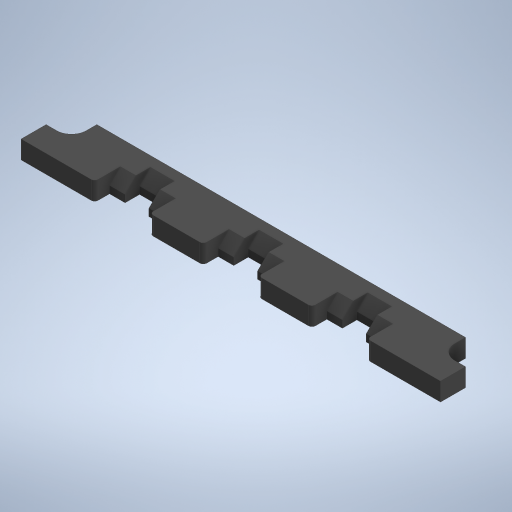
# Autodesk Inventor part: Centreur_resistance
Saved by Autodesk Inventor 2024 (Build 280153000, 153)
## iProperties
Created: 2024-08-30
Part Number: Centreur_resistance
Material: Générique
Document SubType Name: Modeling
Designer: malam
Density: 1 g/cm^3
Appearance: Par défaut
Author: malam
Autodesk Inventor part; units mm, degrees
ref_plane "YZ Plane" through (0, 0, 0) normal (1, 0, 0) x (0, 1, 0)
ref_plane "XZ Plane" through (0, 0, 0) normal (0, 1, 0) x (-1, 0, 0)
ref_plane "XY Plane" through (0, 0, 0) normal (0, 0, 1) x (1, 0, 0)
sketch "Esquisse1" plane through (0, 0, 0) normal (0, 1, 0) x (-1, 0, 0)
  line L0 (60, -42) -> (60, 42)
  line L1 (55, 39) -> (57, 39)
  arc A0 (52, 42) -> (55, 39) centre (55, 42) ccw
  line L2 (52, 44) -> (52, 42)
  line L3 (55, 46) -> (-55, 46)
  circle A1 centre (55, 42.115) radius 2
  arc A2 (60, 42) -> (55, 47) centre (55, 42) ccw
  line L4 (55, 47) -> (-55, 47)
  line L5 (-55, 47) -> (55, 47)
  line L6 (51, 45) -> (-51, 45)
  line L7 (-52, 42) -> (-51, 42)
  arc A3 (-57, 39) -> (-58, 38) centre (-57, 38) ccw
  circle A4 centre (-55, 42.115) radius 2
  line L8 (-55, 39) -> (-55, 38)
  line L9 (-52, 44) -> (-52, 42)
  arc A5 (-51, 45) -> (-52, 44) centre (-51, 44) ccw
  line L10 (-55, 39) -> (-57, 39)
  arc A6 (-55, 39) -> (-52, 42) centre (-55, 42) ccw
  arc A7 (-57, 39) -> (-58, 38) centre (-57, 38) ccw
  circle A8 centre (55, -42.115) radius 2
  line L11 (-55, -39) -> (-57, -39)
  arc A9 (-52, -42) -> (-55, -39) centre (-55, -42) ccw
  line L12 (-52, -44) -> (-52, -42)
  line L13 (52, -42) -> (52, -44)
  circle A10 centre (-55, -42.115) radius 2
  line L14 (-51, -45) -> (51, -45)
  line L15 (51, -45) -> (-51, -45)
  line L16 (-55, -46) -> (55, -46)
  line L17 (-55, -47) -> (55, -47)
  line L18 (55, -47) -> (-55, -47)
  arc A11 (-51, 45) -> (-52, 44) centre (-51, 44) ccw
  line L19 (-52, 42) -> (-52, 44)
  arc A12 (-55, 46) -> (-59, 42) centre (-55, 42) ccw
  line L20 (-51, 42) -> (-51, 45)
  arc A13 (-55, 47) -> (-60, 42) centre (-55, 42) ccw
  circle A14 centre (-55, 42.115) radius 2
  line L21 (-55, 46) -> (-55, 47)
  arc A15 (-55, 47) -> (-60, 42) centre (-55, 42) ccw
  line L22 (52, -42) -> (51, -42)
  arc A16 (51, -45) -> (52, -44) centre (51, -44) ccw
  line L23 (-51, 45) -> (51, 45)
  arc A17 (52, 42) -> (55, 39) centre (55, 42) ccw
  line L24 (55, -39) -> (55, -38)
  line L25 (57, -39) -> (55, -39)
  line L26 (55, -39) -> (57, -39)
  arc A18 (55, -39) -> (52, -42) centre (55, -42) ccw
  arc A19 (57, -39) -> (58, -38) centre (57, -38) ccw
  line L27 (52, -44) -> (52, -42)
  arc A20 (51, -45) -> (52, -44) centre (51, -44) ccw
  circle A21 centre (55, -42.115) radius 2
  arc A22 (57, -39) -> (58, -38) centre (57, -38) ccw
  line L28 (58, 38) -> (58, -38)
  circle A23 centre (55, 42.115) radius 2
  line L29 (52, 42) -> (52, 44)
  line L30 (52, 42) -> (51, 42)
  arc A24 (52, 44) -> (51, 45) centre (51, 44) ccw
  line L31 (55, 39) -> (55, 38)
  arc A25 (52, 44) -> (51, 45) centre (51, 44) ccw
  arc A26 (58, 38) -> (57, 39) centre (57, 38) ccw
  arc A27 (58, 38) -> (57, 39) centre (57, 38) ccw
  line L32 (57, 39) -> (55, 39)
  line L33 (58, -38) -> (58, 38)
  line L34 (58, -38) -> (55, -38)
  line L35 (55, 46) -> (55, 47)
  arc A28 (59, 42) -> (55, 46) centre (55, 42) ccw
  arc A29 (60, 42) -> (55, 47) centre (55, 42) ccw
  line L36 (59, -42) -> (59, 42)
  line L37 (59, 42) -> (60, 42)
  line L38 (60, 42) -> (60, -42)
  line L39 (51, 45) -> (51, 42)
  arc A30 (51, 42) -> (55, 38) centre (55, 42) ccw
  line L40 (55, 38) -> (58, 38)
  arc A31 (55, -39) -> (52, -42) centre (55, -42) ccw
  arc A32 (55, -47) -> (60, -42) centre (55, -42) ccw
  line L41 (-55, -38) -> (-58, -38)
  arc A33 (-51, -42) -> (-55, -38) centre (-55, -42) ccw
  line L42 (-52, -42) -> (-51, -42)
  line L43 (-52, -42) -> (-52, -44)
  line L44 (-51, -45) -> (-51, -42)
  arc A34 (-52, -44) -> (-51, -45) centre (-51, -44) ccw
  circle A35 centre (-55, -42.115) radius 2
  line L45 (-55, -46) -> (-55, -47)
  arc A36 (-59, -42) -> (-55, -46) centre (-55, -42) ccw
  arc A37 (-60, -42) -> (-55, -47) centre (-55, -42) ccw
  line L46 (-60, -42) -> (-59, -42)
  arc A38 (-60, -42) -> (-55, -47) centre (-55, -42) ccw
  arc A39 (-58, -38) -> (-57, -39) centre (-57, -38) ccw
  line L47 (-57, 39) -> (-55, 39)
  arc A40 (-55, 39) -> (-52, 42) centre (-55, 42) ccw
  line L48 (-55, -39) -> (-55, -38)
  line L49 (-58, -38) -> (-58, 38)
  arc A41 (-52, -44) -> (-51, -45) centre (-51, -44) ccw
  arc A42 (-58, -38) -> (-57, -39) centre (-57, -38) ccw
  line L50 (-60, 42) -> (-60, -42)
  arc A43 (-52, -42) -> (-55, -39) centre (-55, -42) ccw
  line L51 (-57, -39) -> (-55, -39)
  line L52 (-58, 38) -> (-58, -38)
  line L53 (-58, 38) -> (-55, 38)
  arc A44 (-55, 38) -> (-51, 42) centre (-55, 42) ccw
  line L54 (-59, 42) -> (-60, 42)
  line L55 (-60, -42) -> (-60, 42)
  line L56 (-59, 42) -> (-59, -42)
  line L57 (55, -46) -> (55, -47)
  arc A45 (55, -38) -> (51, -42) centre (55, -42) ccw
  line L58 (51, -42) -> (51, -45)
  arc A46 (55, -46) -> (59, -42) centre (55, -42) ccw
  line L59 (59, -42) -> (60, -42)
  arc A47 (55, -47) -> (60, -42) centre (55, -42) ccw
  line L60 (-37.5, -35) -> (-22.5, -35)
  line L61 (-37.5, -35) -> (-22.5, -35)
  line L62 (-33.25, 35) -> (-37.5, 35)
  line L63 (-33.25, 35) -> (-31.25, 35)
  line L64 (-31.25, 32) -> (-33.25, 32)
  line L65 (-31.25, 35) -> (-31.25, 32)
  line L66 (-31.25, 32) -> (-33.25, 32)
  line L67 (-28.75, 35) -> (-31.25, 35)
  line L68 (-28.75, 32) -> (-28.75, 35)
  line L69 (-28.75, 32) -> (-28.75, 35)
  line L70 (-26.75, 32) -> (-28.75, 32)
  line L71 (-26.75, 32) -> (-28.75, 32)
  line L72 (-22.5, 35) -> (-37.5, 35)
  line L73 (-22.5, 35) -> (-26.75, 35)
  line L74 (-37.5, 35) -> (-37.5, -35)
  line L75 (-37.5, 35) -> (-37.5, -35)
  line L76 (-22.5, -35) -> (-22.5, 35)
  line L77 (-22.5, -35) -> (-22.5, 35)
  line L78 (-28.75, 35) -> (-26.75, 35)
  line L79 (-31.25, 35) -> (-31.25, 32)
  line L80 (-26.75, 35) -> (-26.75, 32)
  line L81 (-26.75, 35) -> (-26.75, 32)
  line L82 (-33.25, 32) -> (-33.25, 35)
  line L83 (-33.25, 32) -> (-33.25, 35)
  line L84 (-7.5, -35) -> (7.5, -35)
  line L85 (-7.5, -35) -> (7.5, -35)
  line L86 (-3.25, 35) -> (-7.5, 35)
  line L87 (-3.25, 35) -> (-1.25, 35)
  line L88 (-1.25, 32) -> (-3.25, 32)
  line L89 (-1.25, 35) -> (-1.25, 32)
  line L90 (-1.25, 32) -> (-3.25, 32)
  line L91 (1.25, 35) -> (-1.25, 35)
  line L92 (1.25, 32) -> (1.25, 35)
  line L93 (1.25, 32) -> (1.25, 35)
  line L94 (3.25, 32) -> (1.25, 32)
  line L95 (3.25, 32) -> (1.25, 32)
  line L96 (7.5, 35) -> (-7.5, 35)
  line L97 (7.5, 35) -> (3.25, 35)
  line L98 (-7.5, 35) -> (-7.5, -35)
  line L99 (-7.5, 35) -> (-7.5, -35)
  line L100 (7.5, -35) -> (7.5, 35)
  line L101 (7.5, -35) -> (7.5, 35)
  line L102 (1.25, 35) -> (3.25, 35)
  line L103 (-1.25, 35) -> (-1.25, 32)
  line L104 (3.25, 35) -> (3.25, 32)
  line L105 (3.25, 35) -> (3.25, 32)
  line L106 (-3.25, 32) -> (-3.25, 35)
  line L107 (-3.25, 32) -> (-3.25, 35)
  line L108 (22.5, -35) -> (37.5, -35)
  line L109 (22.5, -35) -> (37.5, -35)
  line L110 (26.75, 35) -> (22.5, 35)
  line L111 (26.75, 35) -> (28.75, 35)
  line L112 (28.75, 32) -> (26.75, 32)
  line L113 (28.75, 35) -> (28.75, 32)
  line L114 (28.75, 32) -> (26.75, 32)
  line L115 (31.25, 35) -> (28.75, 35)
  line L116 (31.25, 32) -> (31.25, 35)
  line L117 (31.25, 32) -> (31.25, 35)
  line L118 (33.25, 32) -> (31.25, 32)
  line L119 (33.25, 32) -> (31.25, 32)
  line L120 (37.5, 35) -> (22.5, 35)
  line L121 (37.5, 35) -> (33.25, 35)
  line L122 (22.5, 35) -> (22.5, -35)
  line L123 (22.5, 35) -> (22.5, -35)
  line L124 (37.5, -35) -> (37.5, 35)
  line L125 (37.5, -35) -> (37.5, 35)
  line L126 (31.25, 35) -> (33.25, 35)
  line L127 (28.75, 35) -> (28.75, 32)
  line L128 (33.25, 35) -> (33.25, 32)
  line L129 (33.25, 35) -> (33.25, 32)
  line L130 (26.75, 32) -> (26.75, 35)
  line L131 (26.75, 32) -> (26.75, 35)
  line L132 (55, -42) -> (-55, 42) construction
  line L133 (55, 42) -> (-55, -42) construction
  line L134 (58, -30.8976) -> (-58, -30.8976)
  point P0 (0, 0)
  point P1 (0, 0)
  point P2 (37.5, -30.8976)
  point P3 (22.5, -30.8976)
  point P4 (7.5, -30.8976)
  point P5 (-7.5, -30.8976)
  point P6 (-22.5, -30.8976)
  point P7 (-37.5, -30.8976)
  point P8 (-58, -30.8976)
  constraints: 270 end point, 80 point on circle, 48 centre point, 2 point on line, 1 midpoint, 1 perpendicular
extrude "Extrusion1" add sketch "Esquisse1" along normal blind 5 contours L28 L34 A45 L58 L14 L44 A33 L41 L49 L134 L74 L60 L76 L98 L84 L100 L122 L108 L124
sketch "Esquisse2" plane through (0, 5, 0) normal (0, 1, 0) x (1, 0, 0)
  line L0 (-58, 38) -> (-58, 30.8976) projected
  line L1 (-58, 30.8976) -> (-37.5, 30.8976) projected
  line L2 (-37.5, 30.8976) -> (-37.5, 35) projected
  line L3 (-37.5, 35) -> (-22.5, 35) projected
  line L4 (-22.5, 35) -> (-22.5, 30.8976) projected
  line L5 (-22.5, 30.8976) -> (-7.5, 30.8976) projected
  line L6 (-7.5, 30.8976) -> (-7.5, 35) projected
  line L7 (-7.5, 35) -> (7.5, 35) projected
  line L8 (7.5, 35) -> (7.5, 30.8976) projected
  line L9 (7.5, 30.8976) -> (22.5, 30.8976) projected
  line L10 (22.5, 30.8976) -> (22.5, 35) projected
  line L11 (22.5, 35) -> (37.5, 35) projected
  line L12 (37.5, 35) -> (37.5, 30.8976) projected
  line L13 (37.5, 30.8976) -> (58, 30.8976) projected
  line L14 (58, 30.8976) -> (58, 38) projected
  line L15 (58, 38) -> (55, 38) projected
  arc A0 (51, 42) -> (55, 38) centre (55, 42) ccw projected
  line L16 (51, 42) -> (51, 45) projected
  line L17 (51, 45) -> (-51, 45) projected
  line L18 (-51, 45) -> (-51, 42) projected
  arc A1 (-55, 38) -> (-51, 42) centre (-55, 42) ccw projected
  line L19 (-55, 38) -> (-58, 38) projected
  line L20 (-50.9, 44.9) -> (50.9, 44.9)
  line L21 (50.9, 44.9) -> (50.9, 42)
  arc A2 (50.9, 42) -> (55, 37.9) centre (55, 42) ccw
  line L22 (55, 37.9) -> (57.9, 37.9)
  line L23 (57.9, 37.9) -> (57.9, 30.9976)
  line L24 (57.9, 30.9976) -> (37.6, 30.9976)
  line L25 (37.6, 30.9976) -> (37.6, 35.1)
  line L26 (37.6, 35.1) -> (22.4, 35.1)
  line L27 (22.4, 35.1) -> (22.4, 30.9976)
  line L28 (22.4, 30.9976) -> (7.6, 30.9976)
  line L29 (7.6, 30.9976) -> (7.6, 35.1)
  line L30 (7.6, 35.1) -> (-7.6, 35.1)
  line L31 (-7.6, 35.1) -> (-7.6, 30.9976)
  line L32 (-7.6, 30.9976) -> (-22.4, 30.9976)
  line L33 (-22.4, 30.9976) -> (-22.4, 35.1)
  line L34 (-22.4, 35.1) -> (-37.6, 35.1)
  line L35 (-37.6, 35.1) -> (-37.6, 30.9976)
  line L36 (-37.6, 30.9976) -> (-57.9, 30.9976)
  line L37 (-57.9, 30.9976) -> (-57.9, 37.9)
  line L38 (-57.9, 37.9) -> (-55, 37.9)
  arc A3 (-55, 37.9) -> (-50.9, 42) centre (-55, 42) ccw
  line L39 (-50.9, 42) -> (-50.9, 44.9)
  point P0 (0, 0)
  dimension "d2" = 0.1
  constraints: 40 end point, 4 point on circle, 2 centre point, 21 other
  measures "d2" distance between parallel lines of L17 L20
extrude "Extrusion2" cut sketch "Esquisse2" against normal blind 5
chamfer "Chanfrein1" distance 3 angle 45 3 edges at (-30, 5, -35.1) (0, 5, -35.1) (30, 5, -35.1)
fillet "Congé1" radius 1 6 edges at (-37.6, 2.5, -30.9976) (-22.4, 2.5, -30.9976) (-7.6, 2.5, -30.9976) (7.6, 2.5, -30.9976) (22.4, 2.5, -30.9976) (37.6, 2.5, -30.9976)
sketch "Esquisse4" plane through (0, 5, 0) normal (0, 1, 0) x (1, 0, 0)
  line L0 (-33.3, 31.1) -> (-26.7, 31.1)
  line L1 (-26.7, 31.1) -> (-26.7, 39.1)
  line L2 (-26.7, 39.1) -> (-33.3, 39.1)
  line L3 (-33.3, 39.1) -> (-33.3, 31.1)
  line L4 (-22.4, 35.1) -> (-37.6, 35.1) projected
  line L5 (-33.3, 31.1) -> (-26.7, 39.1) construction
  line L6 (-26.7, 31.1) -> (-33.3, 39.1) construction
  line L7 (-3.3, 31.1) -> (3.3, 31.1)
  line L8 (3.3, 31.1) -> (3.3, 39.1)
  line L9 (3.3, 39.1) -> (-3.3, 39.1)
  line L10 (-3.3, 39.1) -> (-3.3, 31.1)
  line L11 (7.6, 35.1) -> (-7.6, 35.1) projected
  line L12 (-3.3, 31.1) -> (3.3, 39.1) construction
  line L13 (3.3, 31.1) -> (-3.3, 39.1) construction
  line L14 (26.7, 31.1) -> (33.3, 31.1)
  line L15 (33.3, 31.1) -> (33.3, 39.1)
  line L16 (33.3, 39.1) -> (26.7, 39.1)
  line L17 (26.7, 39.1) -> (26.7, 31.1)
  line L18 (37.6, 35.1) -> (22.4, 35.1) projected
  line L19 (26.7, 31.1) -> (33.3, 39.1) construction
  line L20 (33.3, 31.1) -> (26.7, 39.1) construction
  point P0 (0, 0)
  point P1 (-30, 35.1)
  point P2 (0, 35.1)
  point P3 (30, 35.1)
  point P4 (26.7, 35.1)
  point P5 (33.3, 35.1)
  point P6 (-3.3, 35.1)
  point P7 (3.3, 35.1)
  point P8 (-33.3, 35.1)
  point P9 (-26.7, 35.1)
  dimension "d9" = 6.6
  dimension "d10" = 8
  dimension "d11" = 6.6
  dimension "d12" = 8
  dimension "d13" = 6.6
  constraints: 36 end point, 9 midpoint, 6 parallel, 3 horizontal, 3 perpendicular, 1 point on line
  measures "d9" distance of L2.end L1.end
  measures "d10" distance of L1.end L0.end
  measures "d11" distance of L9.end L8.end
  measures "d12" distance of L8.end L7.end
  measures "d13" distance of L16.end L15.end
extrude "Extrusion3" cut sketch "Esquisse4" against normal blind 5 contours L3 L2 L1 L4 | L10 L9 L8 L11 | L17 L16 L15 L18
chamfer "Chanfrein2" distance 3 angle 45 3 edges at (-30, 5, -39.1) (0, 5, -39.1) (30, 5, -39.1)
